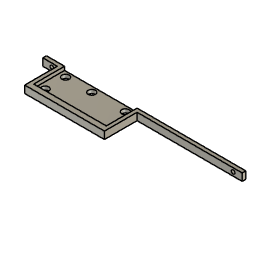
Suporte do botão v1 (Autodesk Fusion 360 design; units mm, degrees)
Autodesk Fusion 360 part; units mm, degrees
sketch "Esboço1" plane through (0, 0, 0) normal (0, 0, 1) x (1, 0, 0)
  line L0 (0, 0) -> (110, 0)
  line L1 (110, 0) -> (110, -5)
  line L2 (55, -20) -> (5, -20)
  line L3 (0, -5) -> (0, 0)
  line L4 (0, 0) -> (55, 0)
  line L5 (0, -5) -> (0, 0)
  line L6 (35, 0) -> (75, 0)
  line L7 (0, 0) -> (10, 0)
  line L8 (10, 0) -> (10, -10)
  line L9 (0, -5) -> (0, 0)
  line L10 (10, 0) -> (50, 0)
  line L11 (50, 0) -> (50, -17)
  line L12 (50, -17) -> (10, -17)
  line L13 (10, -17) -> (10, 0)
  line L14 (10, 0) -> (50, 0)
  line L15 (50, 0) -> (50, -17)
  line L16 (50, -17) -> (10, -17)
  line L17 (10, -17) -> (10, 0)
  circle A0 centre (46.5001, -2.9491) radius 2
  circle A1 centre (46.5001, -14.1881) radius 2
  circle A2 centre (30, -14.1881) radius 2
  line L18 (30, -12.1881) -> (30, -17)
  circle A3 centre (13.4999, -14.1881) radius 2
  line L19 (0, 0) -> (5, 0)
  line L20 (0, -5) -> (0, 0)
  line L21 (110, 0) -> (105, 0)
  line L22 (110, -5) -> (110, 0)
  line L23 (55, -20) -> (110, -5)
  line L24 (5, -20) -> (0, -5)
  line L25 (0, 0) -> (5, 0)
  line L26 (5, 0) -> (5, 5)
  line L27 (5, 5) -> (0, 5)
  line L28 (0, 5) -> (0, 0)
  line L29 (105, 0) -> (110, 0)
  line L30 (110, 0) -> (110, 5)
  line L31 (110, 5) -> (105, 5)
  line L32 (105, 5) -> (105, 0)
  dimension "d1" = 110
  dimension "d3" = 55
  dimension "d5" = 40
  dimension "d7" = 40
  dimension "d8" = 17
  dimension "d9" = 40
  dimension "d10" = 17
  dimension "d11" = 4
  dimension "d12" = 4
  dimension "d13" = 4
  dimension "d14" = 5
  dimension "d15" = 5
  dimension "d16" = 5
  dimension "d17" = 5
  constraint horizontal L0
  constraint vertical L1
  constraint horizontal L2
  constraint vertical L3
  constraint coincident L0.start L3.end
  constraint horizontal L4
  constraint vertical L5
  constraint horizontal L6
  constraint coincident L4 L6.start
  constraint horizontal L7
  constraint vertical L8
  constraint vertical L9
  constraint horizontal L10
  constraint vertical L11
  constraint horizontal L12
  constraint vertical L13
  constraint horizontal L14
  constraint vertical L15
  constraint horizontal L16
  constraint vertical L17
  constraint vertical A0.centre A1.centre
  constraint horizontal A1.centre A2.centre
  constraint midpoint L12 L18.end
  constraint symmetric A1 L18 A3
  constraint coincident A2 L18.start
  constraint horizontal L19
  constraint vertical L20
  constraint horizontal L21
  constraint vertical L22
  constraint horizontal L25
  constraint vertical L26
  constraint horizontal L27
  constraint vertical L28
  constraint horizontal L29
  constraint vertical L30
  constraint horizontal L31
  constraint vertical L32
  measures "d1" distance of L0.start L0.end
  measures "d3" distance of L0.start L4.end
  measures "d5" distance of L6.start L6.end
  measures "d7" distance of L7.end L10.end
  measures "d8" distance of L7.end L12.end
  measures "d9" distance of L7.end L10.end
  measures "d10" distance of L7.end L12.end
  measures "d11" diameter of A0
  measures "d12" diameter of A1
  measures "d13" diameter of A2
  measures "d14" distance of L0.start L19.end
  measures "d15" distance of L0.start L3.start
  measures "d16" distance of L0.end L21.end
  measures "d17" distance of L0.end L1.end
extrude "Extrusão1" add sketch "Esboço1" along normal blind 2 contours L0 L4 L6 L8 L10 L11 L12 L13 L14 L15 L16 L17
extrude "Extrusão2" add sketch "Esboço1" along normal blind 4 contours L0 L1 L2 L3 L4 L5 L6 L7 L8 L9 L11 L12 L13 L15 L16 L17 L19 L20 L21 L22 L23 L24 L25 L29
extrude "Extrusão3" add sketch "Esboço1" along normal blind 1 contours L0 L21 L29 L30 L31 L32
extrude "Extrusão4" add sketch "Esboço1" along normal blind 1 contours L0 L4 L7 L19 L25 L26 L27 L28
sketch "Esboço2" plane through (0, 5, 0) normal (0, 1, 0) x (-1, 0, 0)
  line L0 (-110, 0) -> (-105, 0)
  line L1 (-105, 0) -> (-105, 1)
  line L2 (-105, 1) -> (-110, 1)
  line L3 (-110, 1) -> (-110, 0)
  circle A0 centre (-105, 2) radius 1
  circle A1 centre (-5, 2) radius 1
  dimension "d26" = 2
  measures "d26" diameter of A0
hole "Furo1" at (105, 5, 2) direction (0, -1, 0) diameter 2 depth 38 tip angle 118
hole "Furo2" at (5, 5, 2) direction (0, -1, 0) diameter 2 depth 38 tip angle 118
sketch "Esboço3" plane through (0, 0, 0) normal (0, 0, 1) x (1, 0, 0)
  line L0 (0, 0) -> (10, 0)
  line L1 (10, 0) -> (10, -2)
  line L2 (10, -2) -> (0, -2)
  line L3 (0, -2) -> (0, 0)
  line L4 (7, 0) -> (10, 0)
  line L5 (10, 0) -> (10, -20)
  line L6 (10, -20) -> (7, -20)
  line L7 (7, -20) -> (7, 0)
  line L8 (10, -20) -> (7, -20)
  line L9 (7, -20) -> (7, -2)
  line L10 (7, -2) -> (10, -2)
  line L11 (10, -2) -> (10, -20)
  line L12 (7, -20) -> (5, -20)
  line L13 (5, -20) -> (5, -2)
  line L14 (5, -2) -> (7, -2)
  line L15 (7, -2) -> (7, -20)
  dimension "d33" = 2
  constraint horizontal L0
  constraint vertical L1
  constraint horizontal L2
  constraint vertical L3
  constraint coincident L0.start L3.end
  constraint horizontal L4
  constraint vertical L5
  constraint horizontal L6
  constraint vertical L7
  constraint coincident L0 L4.start
  constraint horizontal L8
  constraint vertical L9
  constraint horizontal L10
  constraint vertical L11
  constraint coincident L2 L9.end
  constraint coincident L7 L9.end
  constraint horizontal L12
  constraint vertical L13
  constraint horizontal L14
  constraint vertical L15
  constraint midpoint L2 L13.end
  measures "d33" distance of L0.start L2.end
sketch "Esboço4" plane through (0, 0, 0) normal (0, 0, 1) x (1, 0, 0)
  line L0 (8, 0) -> (10, 0)
  line L1 (10, 0) -> (10, -20)
  line L2 (10, -20) -> (8, -20)
  line L3 (8, -20) -> (8, 0)
  line L4 (10, 0) -> (0, 0)
  line L5 (0, 0) -> (0, -2)
  line L6 (0, -2) -> (10, -2)
  line L7 (10, -2) -> (10, 0)
  line L8 (8, -20) -> (0, -20)
  line L9 (0, -20) -> (0, -2)
  line L10 (0, -2) -> (8, -2)
  line L11 (8, -2) -> (8, -20)
  constraint horizontal L0
  constraint vertical L1
  constraint horizontal L2
  constraint vertical L3
  constraint horizontal L4
  constraint vertical L5
  constraint horizontal L6
  constraint vertical L7
  constraint horizontal L8
  constraint vertical L9
  constraint horizontal L10
  constraint vertical L11
extrude "Extrusão6" cut sketch "Esboço4" along normal blind 2 contours L3 L6 L8 L9 L10 L11
extrude "Extrusão7" cut sketch "Esboço4" along normal blind 4 contours L3 L6 L8 L9 L10 L11
sketch "Esboço5" plane through (0, 0, 0) normal (0, 0, 1) x (1, 0, 0)
  line L0 (52, -20) -> (110, -20)
  line L1 (110, -20) -> (110, -2)
  line L2 (110, -2) -> (52, -2)
  line L3 (52, -2) -> (52, -20)
  constraint horizontal L0
  constraint vertical L1
  constraint horizontal L2
  constraint vertical L3
extrude "Extrusão8" cut sketch "Esboço5" along normal blind 4
extrude "Extrusão9" cut 1 faces at (108.3333, 1.6667, 1) along direction (0, 0, -1) blind 1
extrude "Extrusão10" cut 1 faces at (1.6667, 3.3333, 1) along direction (0, 0, -1) blind 1
sketch "Esboço6" plane through (0, 0, 0) normal (0, 0, 1) x (1, 0, 0)
  circle A0 centre (13.4999, -2.9491) radius 2
  point P0 (13.4999, -14.1881)
  point P1 (46.5001, -2.9491)
  dimension "d46" = 4
  constraint vertical A0.centre P0
  constraint horizontal A0.centre P1
  measures "d46" diameter of A0
extrude "Extrusão14" cut sketch "Esboço6" along normal blind 2
sketch "Esboço7" plane through (0, 0, 0) normal (0, 0, 1) x (1, 0, 0)
  circle A0 centre (27.9799, -2.9491) radius 2
  point P0 (13.4999, -2.9491)
  dimension "d55" = 4
  constraint horizontal A0.centre P0
  measures "d55" diameter of A0
extrude "Extrusão15" cut sketch "Esboço7" along normal blind 2
extrude "Extrusão16" add sketch "Esboço1" along normal blind 2 contours A1 | A2 L18 picked at (28.599, -14.3364)
extrude "Extrusão17" add sketch "Esboço1" along normal blind 2 contours A2 L18 picked at (31.4707, -14.5893)
